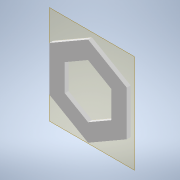
# Autodesk Inventor part: Electrical
Saved by Autodesk Inventor 2020.3 (Build 243373000, 373)
## iProperties
Created: 2020-07-07
Part Number: Electrical
Material: Acetal Resin, Black
Document SubType Name: Modeling
Designer: Bruno
Density: 1.425 g/cm^3
Appearance: Smooth - Black
Author: Bruno
Autodesk Inventor part; units mm, degrees
ref_plane "YZ Plane" through (0, 0, 0) normal (1, 0, 0) x (0, 1, 0)
ref_plane "XZ Plane" through (0, 0, 0) normal (0, 1, 0) x (-1, 0, 0)
ref_plane "XY Plane" through (0, 0, 0) normal (0, 0, 1) x (1, 0, 0)
ref_plane "Work Plane1" through (0, 0, 0) normal (0, 0, 1) x (1, 0, 0)
sketch "Sketch1" plane through (0, 0, 0) normal (0, 0, 1) x (1, 0, 0)
  line L0 (498, -287.5204) -> (0, -575.0409)
  line L1 (0, -575.0409) -> (-498, -287.5204)
  line L2 (-498, -287.5204) -> (-498, 287.5204)
  line L3 (-498, 287.5204) -> (0, 575.0409)
  line L4 (0, 575.0409) -> (498, 287.5204)
  line L5 (498, 287.5204) -> (498, -287.5204)
  line L6 (300, -173.2051) -> (0, -346.4102)
  line L7 (0, -346.4102) -> (-300, -173.2051)
  line L8 (-300, -173.2051) -> (-300, 173.2051)
  line L9 (-300, 173.2051) -> (0, 346.4102)
  line L10 (0, 346.4102) -> (300, 173.2051)
  line L11 (300, 173.2051) -> (300, -173.2051)
  point P0 (0, 0)
  point P1 (0, 0)
  point P2 (0, 0)
  dimension "d0" = 300
  dimension "d1" = 498
  constraints: 24 end point, 2 coincident, 2 vertical, 26 other
  measures "d0" distance from line of point (0, 0) L11
  measures "d1" distance from line of point (0, 0) L5
extrude "Extrusion1" add sketch "Sketch1" along normal blind 50
body "Solid1"
